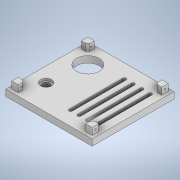
# Autodesk Inventor part: GameFrameRaspiBox2
Saved by Autodesk Inventor 2022 (Build 260153000, 153)
## iProperties
Created: 2022-03-27
Part Number: GameFrameRaspiBox2
Material: Generisch
Document SubType Name: Modeling
Designer: Max
Density: 1 g/cm^3
Appearance: Vorgabe
Author: Max
Autodesk Inventor part; units mm, degrees
ref_plane "YZ Plane" through (0, 0, 0) normal (1, 0, 0) x (0, 1, 0)
ref_plane "XZ Plane" through (0, 0, 0) normal (0, 1, 0) x (-1, 0, 0)
ref_plane "XY Plane" through (0, 0, 0) normal (0, 0, 1) x (1, 0, 0)
sketch "Skizze1" plane through (0, 0, 0) normal (0, 1, 0) x (-1, 0, 0)
  line L0 (23.4402, 37.0701) -> (-56.5598, 37.0701)
  line L1 (-56.5598, 37.0701) -> (-56.5598, -38.9299)
  line L2 (-56.5598, -38.9299) -> (23.4402, -38.9299)
  line L3 (23.4402, -38.9299) -> (23.4402, 37.0701)
  point P0 (0, 0)
  dimension "d0" = 76
  dimension "d1" = 80
  constraints: 8 end point, 2 parallel, 1 horizontal, 1 perpendicular
  measures "d0" distance of L2.end L0.start
  measures "d1" distance of L0.start L0.end
extrude "Extrusion1" add sketch "Skizze1" along normal blind 6
sketch "Skizze8" plane through (0, 0, 0) normal (0, -1, 0) x (1, 0, 0)
  line L0 (47.5598, 24.0701) -> (47.5598, -25.9299) construction
  line L1 (49.0598, 24.0701) -> (49.0598, -25.9299)
  line L2 (46.0598, -25.9299) -> (46.0598, 24.0701)
  arc A0 (49.0598, 24.0701) -> (46.0598, 24.0701) centre (47.5598, 24.0701) ccw
  arc A1 (46.0598, -25.9299) -> (49.0598, -25.9299) centre (47.5598, -25.9299) ccw
  line L3 (52.5598, -0.9299) -> (-23.4402, -0.9299)
  line L4 (39.5598, 24.0701) -> (39.5598, -25.9299) construction
  line L5 (38.0598, 24.0701) -> (38.0598, -25.9299)
  line L6 (41.0598, -25.9299) -> (41.0598, 24.0701)
  arc A2 (41.0598, 24.0701) -> (38.0598, 24.0701) centre (39.5598, 24.0701) ccw
  arc A3 (38.0598, -25.9299) -> (41.0598, -25.9299) centre (39.5598, -25.9299) ccw
  line L7 (56.5598, 37.0701) -> (56.5598, -38.9299) projected
  line L8 (56.5598, -38.9299) -> (-23.4402, -38.9299) projected
  line L9 (41.0598, 24.0701) -> (38.0598, 24.0701) construction
  line L10 (41.0598, -25.9299) -> (38.0598, -25.9299) construction
  line L11 (49.0598, -25.9299) -> (46.0598, -25.9299) construction
  arc A4 (30.0598, -25.9299) -> (33.0598, -25.9299) centre (31.5598, -25.9299) ccw
  line L12 (31.5598, 24.0701) -> (31.5598, -25.9299) construction
  line L13 (30.0598, 24.0701) -> (30.0598, -25.9299)
  line L14 (33.0598, -25.9299) -> (33.0598, 24.0701)
  arc A5 (33.0598, 24.0701) -> (30.0598, 24.0701) centre (31.5598, 24.0701) ccw
  line L15 (33.0598, 24.0701) -> (30.0598, 24.0701) construction
  line L16 (33.0598, -25.9299) -> (30.0598, -25.9299) construction
  line L17 (25.0598, 24.0701) -> (22.0598, 24.0701) construction
  arc A6 (25.0598, 24.0701) -> (22.0598, 24.0701) centre (23.5598, 24.0701) ccw
  line L18 (25.0598, -25.9299) -> (25.0598, 24.0701)
  line L19 (23.5598, 24.0701) -> (23.5598, -25.9299) construction
  line L20 (22.0598, 24.0701) -> (22.0598, -25.9299)
  line L21 (25.0598, -25.9299) -> (22.0598, -25.9299) construction
  arc A7 (22.0598, -25.9299) -> (25.0598, -25.9299) centre (23.5598, -25.9299) ccw
  circle A8 centre (-9.8402, 13.4701) radius 3.6
  line L22 (-23.4402, 37.0701) -> (56.5598, 37.0701) projected
  line L23 (-23.4402, -38.9299) -> (-23.4402, 37.0701) projected
  circle A9 centre (-4.9402, -20.4299) radius 10.5
  point P0 (47.5598, -0.9299)
  point P1 (35.0598, -0.9299)
  dimension "d69" = 7.5
  dimension "d70" = 50
  dimension "d71" = 38
  dimension "d72" = 5
  dimension "d74" = 3
  dimension "d75" = 5
  dimension "d76" = 5
  dimension "d77" = 7.2
  dimension "d78" = 23.6
  dimension "d79" = 13.6
  dimension "d109" = 21
  dimension "d110" = 18.5
  dimension "d111" = 18.5
  constraints: 48 end point, 16 point on circle, 10 centre point, 8 horizontal, 7 midpoint, 6 equal length, 4 parallel, 4 tangent, 1 point on line, 1 vertical, 4 other
  measures "d70" distance of L1.start L1.end
  measures "d71" distance between parallel lines of L8 L3
  measures "d72" distance between parallel lines of L2 L6
  measures "d74" distance of L1.end L2.start
  measures "d75" distance between parallel lines of L5 L14
  measures "d76" distance between parallel lines of L13 L18
  measures "d77" diameter of A8
  measures "d78" distance from line of L22 A8.centre
  measures "d79" distance from line of L23 A8.centre
  measures "d109" diameter of A9
  measures "d110" distance from line of L23 A9.centre
  measures "d111" distance from line of L8 A9.centre
extrude "Extrusion8" cut sketch "Skizze8" against normal blind 10 contours L1 L3 L2 A0 | L1 A1 L2 L3 | L6 A3 L5 L3 | L3 L5 A2 L6 | L14 A4 L13 L3 | L3 L13 A5 L14 | L18 A7 L20 L3 | L3 L20 A6 L18 | A8 | A9
sketch "Skizze13" plane through (0, 6, 0) normal (0, 1, 0) x (1, 0, 0)
  circle A0 centre (-9.8402, -13.4701) radius 5.1
  circle A1 centre (-9.8402, -13.4701) radius 3.6 projected
  dimension "d80" = 10.2
  constraints: 1 centre point, 1 coincident
  measures "d80" diameter of A0
extrude "Extrusion13" cut sketch "Skizze13" against normal blind 2
sketch "Skizze14" plane through (0, 6, 0) normal (0, 1, 0) x (1, 0, 0)
  line L0 (-20.7402, -34.3701) -> (-14.7402, -34.3701)
  line L1 (-14.7402, -34.3701) -> (-14.7402, -28.3701)
  line L2 (-14.7402, -28.3701) -> (-20.7402, -28.3701)
  line L3 (-20.7402, -28.3701) -> (-20.7402, -34.3701)
  line L4 (-20.7402, 36.2299) -> (-14.7402, 36.2299)
  line L5 (-14.7402, 36.2299) -> (-14.7402, 30.2299)
  line L6 (-14.7402, 30.2299) -> (-20.7402, 30.2299)
  line L7 (-20.7402, 30.2299) -> (-20.7402, 36.2299)
  line L8 (-23.4402, 38.9299) -> (-23.4402, -37.0701) projected
  line L9 (56.5598, 38.9299) -> (-23.4402, 38.9299) projected
  line L10 (-23.4402, -37.0701) -> (56.5598, -37.0701) projected
  line L11 (47.8598, 30.2299) -> (53.8598, 30.2299)
  line L12 (53.8598, 30.2299) -> (53.8598, 36.2299)
  line L13 (53.8598, 36.2299) -> (47.8598, 36.2299)
  line L14 (47.8598, 36.2299) -> (47.8598, 30.2299)
  line L15 (53.8598, -34.3701) -> (47.8598, -34.3701)
  line L16 (47.8598, -34.3701) -> (47.8598, -28.3701)
  line L17 (47.8598, -28.3701) -> (53.8598, -28.3701)
  line L18 (53.8598, -28.3701) -> (53.8598, -34.3701)
  line L19 (56.5598, -37.0701) -> (56.5598, 38.9299) projected
  point P0 (0, 0)
  dimension "d79" = 13.6
  dimension "d83" = 6
  dimension "d84" = 2.7
  dimension "d85" = 2.7
  dimension "d86" = 2.7
  dimension "d112" = 2.7
  constraints: 32 end point, 8 parallel, 7 equal length, 4 collinear, 4 horizontal, 4 perpendicular
  measures "d83" distance of L4.start L4.end
  measures "d84" distance between parallel lines of L8 L7
  measures "d85" distance between parallel lines of L9 L4
  measures "d86" distance between parallel lines of L10 L0
  measures "d112" distance between parallel lines of L19 L18
extrude "Extrusion14" add sketch "Skizze14" along normal blind 6.5 contours L3 L2 L1 L0 | L4 L5 L6 L7 | L14 L13 L12 L11 | L15 L16 L17 L18
sketch "Skizze17" plane through (-20.7402, 6, -36.2299) normal (-1, 0, 0) x (0, 0, 1)
  circle A0 centre (67.6, 3.25) radius 0.75
  circle A1 centre (3, 3.25) radius 0.75
  line L0 (-2.7, 0) -> (73.3, 0) projected
  line L1 (0, 0) -> (0, 6.5) projected
  line L2 (70.6, 0) -> (70.6, 6.5) projected
  point P0 (36.2299, -6)
  dimension "d102" = 3.25
  dimension "d103" = 1.5
  dimension "d104" = 3
  dimension "d105" = 3
  dimension "d106" = 3.25
  constraints: 2 centre point, 1 equal radius
  measures "d102" distance from line of L0 A1.centre
  measures "d103" diameter of A1
  measures "d104" distance from line of L1 A1.centre
  measures "d105" distance from line of L2 A0.centre
  measures "d106" distance from line of L0 A0.centre
extrude "Extrusion17" cut sketch "Skizze17" against normal through all
chamfer "Fase1" distance 2 angle 45 4 edges at (-14.7402, 9.25, 28.3701) (-14.7402, 9.25, -30.2299) (47.8598, 9.25, 28.3701) (47.8598, 9.25, -30.2299)
